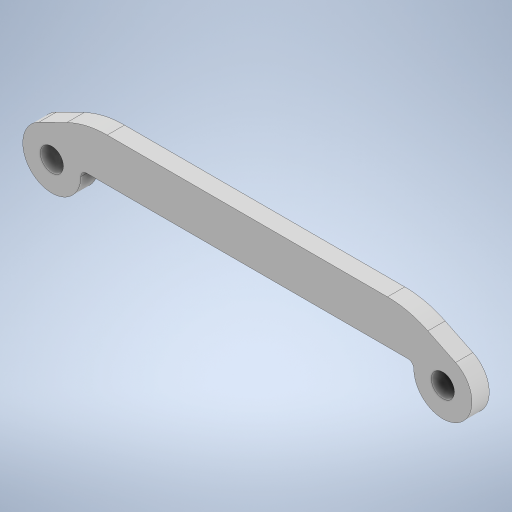
# Autodesk Inventor part: Front Lower arm Brace
Saved by Autodesk Inventor 2024 (Build 280153000, 153)
## iProperties
Created: 2023-07-03
Part Number: Front Lower arm Brace
Material: Generic
Document SubType Name: Modeling
Designer: patel
Density: 1 g/cm^3
Appearance: Default
Author: patel
Autodesk Inventor part; units mm, degrees
ref_plane "YZ Plane" through (0, 0, 0) normal (1, 0, 0) x (0, 1, 0)
ref_plane "XZ Plane" through (0, 0, 0) normal (0, 1, 0) x (-1, 0, 0)
ref_plane "XY Plane" through (0, 0, 0) normal (0, 0, 1) x (1, 0, 0)
sketch "Sketch1" plane through (0, 0, 0) normal (0, 0, 1) x (1, 0, 0)
  line L0 (-22.225, 0) -> (22.225, 0)
  line L1 (-22.225, 0) -> (-28.6752, -3.1405)
  arc A0 (-28.6752, -3.1405) -> (-22.9235, -6.7373) centre (-26.924, -6.7374) ccw
  line L2 (-22.9235, -6.7373) -> (-22.9235, -5.9627)
  circle A1 centre (-26.924, -6.7374) radius 1.5875
  line L3 (0, 2.4501) -> (0, -14.7004) construction
  line L4 (22.225, 0) -> (28.6752, -3.1405)
  arc A2 (22.9235, -6.7373) -> (28.6752, -3.1405) centre (26.924, -6.7374) ccw
  circle A3 centre (26.924, -6.7374) radius 1.5875
  line L5 (22.9235, -6.7373) -> (22.9235, -5.9627)
  line L6 (-22.9235, -5.9627) -> (22.9235, -5.9627)
  point P0 (0, 0)
  point P1 (0, 0)
  point P2 (-26.924, -10.7378)
  point P3 (-22.9235, -6.35)
  dimension "d0" = 44.45
  dimension "d1" = 4.0005
  dimension "d2" = 3.175
  dimension "d3" = 4.7752
  dimension "d4" = 6.35
  dimension "d5" = 26.924
  constraints: 12 end point, 5 point on circle, 5 symmetric about line, 4 centre point, 3 coincident, 2 horizontal, 2 midpoint, 2 tangent, 1 perpendicular, 2 other
  measures "d0" distance of L0.start L0.end
  measures "d1" radius of A0
  measures "d2" diameter of A1
  measures "d3" vertical distance of point (-26.924, -10.738) L2.end
  measures "d4" distance from line of L0 point (-22.924, -6.35)
  measures "d5" distance from line of L3 A0.centre
extrude "Extrusion1" add sketch "Sketch1" along normal mid plane 2.3813
fillet "Fillet1" radius 12.7 2 edges at (-22.225, 0, 0) (22.225, 0, 0)
fillet "Fillet2" radius 0.8128 2 edges at (-22.9235, -5.9627, 0) (22.9235, -5.9627, 0)
body "Solid1"
